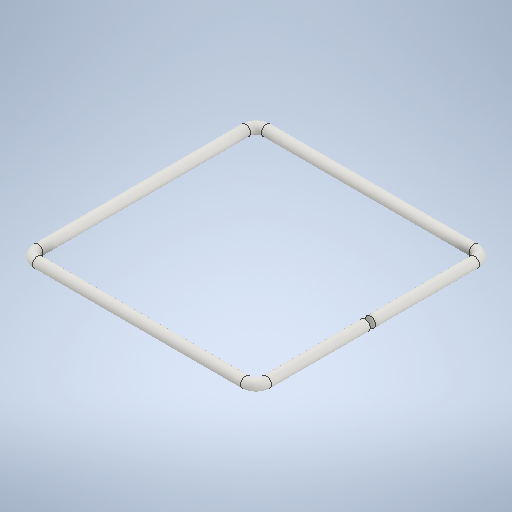
# Autodesk Inventor part: Ring_Of_Rebar
Saved by Autodesk Inventor 2025 (Build 290162010, 162A)
## iProperties
Created: 2024-09-07
Part Number: Ring_Of_Rebar
Material: Steel
Document SubType Name: Modeling
Designer: Tom
Density: 7.85 g/cm^3
Appearance: Steel
Author: Tom
Autodesk Inventor part; units mm, degrees
ref_plane "YZ Plane" through (0, 0, 0) normal (1, 0, 0) x (0, 1, 0)
ref_plane "XZ Plane" through (0, 0, 0) normal (0, 1, 0) x (-1, 0, 0)
ref_plane "XY Plane" through (0, 0, 0) normal (0, 0, 1) x (1, 0, 0)
sketch "Sketch1" plane through (0, 0, 0) normal (0, 0, 1) x (1, 0, 0)
  circle A0 centre (0, 0) radius 6.35
  dimension "d0" = 12.7
  constraints: 1 centre point, 1 coincident
  measures "d0" diameter of A0
sketch "Sketch2" plane through (0, 0, 0) normal (0, 1, 0) x (-1, 0, 0)
  line L0 (0, 0) -> (0, -127)
  line L1 (12.7, -139.7) -> (266.7, -139.7)
  line L2 (279.4, -127) -> (279.4, 127)
  line L3 (266.7, 139.7) -> (12.7, 139.7)
  line L4 (0, 127) -> (0, 6.35)
  arc A0 (0, -127) -> (12.7, -139.7) centre (12.7, -127) ccw
  arc A1 (266.7, -139.7) -> (279.4, -127) centre (266.7, -127) ccw
  arc A2 (279.4, 127) -> (266.7, 139.7) centre (266.7, 127) ccw
  arc A3 (12.7, 139.7) -> (0, 127) centre (12.7, 127) ccw
  point P0 (0, -139.7)
  point P1 (279.4, -139.7)
  point P2 (279.4, 139.7)
  point P3 (0, 139.7)
  dimension "d1" = 6.35
  dimension "d2" = 139.7
  dimension "d3" = 279.4
  dimension "d4" = 279.4
  dimension "d8" = 12.7
  constraints: 10 end point, 10 point on line, 8 point on circle, 8 tangent, 4 centre point, 3 equal radius, 2 perpendicular, 1 parallel, 1 vertical
  measures "d1" distance of L4.end L0.start
  measures "d2" distance of L0.start point (0, -139.7)
  measures "d3" distance of point (0, -139.7) point (279.4, -139.7)
  measures "d4" distance of point (279.4, -139.7) point (279.4, 139.7)
  measures "d8" radius of A0
sweep "Sweep1" add profiles "Sketch1" path "Sketch2" path curves L0 A0 L1 A1 L2 A2 L3 A3 L4
body "Solid1"
